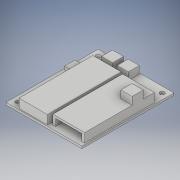
# Autodesk Inventor part: PCB
Saved by Autodesk Inventor 2017 (Build 210142000, 142)
## iProperties
Created: 2017-03-19
Part Number: PCB
Material: Generic
Document SubType Name: Modeling
Designer: Liam
Density: 1 g/cm^3
Appearance: Default
Author: Liam
Autodesk Inventor part; units mm, degrees
ref_plane "YZ Plane" through (0, 0, 0) normal (1, 0, 0) x (0, 1, 0)
ref_plane "XZ Plane" through (0, 0, 0) normal (0, 1, 0) x (-1, 0, 0)
ref_plane "XY Plane" through (0, 0, 0) normal (0, 0, 1) x (1, 0, 0)
sketch "Sketch1" plane through (0, 0, 0) normal (0, 1, 0) x (-1, 0, 0)
  line L0 (0, 0) -> (-54.5338, 0)
  line L1 (-54.5338, 0) -> (-54.5338, -66.1924)
  line L2 (-54.5338, -66.1924) -> (0, -66.1924)
  line L3 (0, -66.1924) -> (0, 0)
  dimension "d0" = 54.5338
  dimension "d1" = 66.1924
  constraints: 8 end point, 2 parallel, 1 horizontal, 1 perpendicular
  measures "d0" distance of L2.end L1.end
  measures "d1" distance of L1.end L0.end
extrude "Extrusion1" add sketch "Sketch1" along normal blind 1.5875
sketch "Sketch2" plane through (0, 1.5875, 0) normal (0, 1, 0) x (1, 0, 0)
  line L0 (0, 66.1924) -> (0, 0) projected
  line L1 (54.5338, 66.1924) -> (0, 66.1924) projected
  line L2 (54.5338, 0) -> (54.5338, 66.1924) projected
  line L3 (0, 0) -> (54.5338, 0) projected
  point P0 (4.3434, 61.7982)
  point P1 (50.419, 61.849)
  point P2 (4.0894, 4.4196)
  dimension "d4" = 4.3434
  dimension "d5" = 4.3942
  dimension "d6" = 4.1148
  dimension "d7" = 4.3434
  dimension "d8" = 4.0894
  dimension "d9" = 4.4196
  measures "d4" distance from line of L0 point (4.343, 61.798)
  measures "d5" distance from line of point (4.343, 61.798) L1
  measures "d6" distance from line of point (50.419, 61.849) L2
  measures "d7" distance from line of point (50.419, 61.849) L1
  measures "d8" distance from line of point (4.089, 4.42) L0
  measures "d9" distance from line of L3 point (4.089, 4.42)
hole "Hole1" at (4.3434, 1.5875, -61.7982) at (50.419, 1.5875, -61.849) at (4.0894, 1.5875, -4.4196) direction (0, -1, 0) diameter 3.175 end through all
sketch "Sketch3" plane through (0, 1.5875, 0) normal (0, 1, 0) x (1, 0, 0)
  line L0 (53.721, 52.8828) -> (53.721, 2.8448)
  line L1 (30.861, 2.8448) -> (30.861, 52.8828)
  line L2 (0, 0) -> (54.5338, 0) projected
  line L3 (54.5338, 0) -> (54.5338, 66.1924) projected
  line L4 (32.893, 52.8828) -> (32.893, 2.8448)
  line L5 (51.689, 52.8828) -> (51.689, 2.8448)
  line L6 (30.861, 52.8828) -> (32.893, 52.8828)
  line L7 (51.689, 52.8828) -> (53.721, 52.8828)
  line L8 (53.721, 2.8448) -> (51.689, 2.8448)
  line L9 (32.893, 2.8448) -> (30.861, 2.8448)
  dimension "d17" = 22.86
  dimension "d18" = 50.038
  dimension "d20" = 0.8128
  dimension "d21" = 2.032
  dimension "d22" = 2.032
  constraints: 16 end point, 6 perpendicular, 5 parallel, 2 horizontal
  measures "d17" distance of L0.end L1.start
  measures "d18" distance of L0.start L0.end
  measures "d20" distance between parallel lines of L3 L0
  measures "d21" distance between parallel lines of L4 L1
  measures "d22" distance between parallel lines of L5 L0
extrude "Extrusion2" add sketch "Sketch3" along normal blind 5
sketch "Sketch4" plane through (0, 6.5875, 0) normal (0, 1, 0) x (1, 0, 0)
  line L0 (30.861, 52.8828) -> (30.861, 2.8448) projected
  line L1 (30.861, 2.8448) -> (32.893, 2.8448) projected
  line L2 (32.893, 2.8448) -> (32.893, 52.8828) projected
  line L3 (32.893, 52.8828) -> (30.861, 52.8828) projected
  line L4 (53.721, 2.8448) -> (53.721, 52.8828) projected
  line L5 (51.689, 52.8828) -> (51.689, 2.8448) projected
  line L6 (51.689, 2.8448) -> (53.721, 2.8448) projected
  line L7 (53.721, 52.8828) -> (51.689, 52.8828) projected
  line L8 (30.861, 52.8828) -> (30.861, 2.8448) projected
  line L9 (30.861, 52.8828) -> (53.721, 52.8828)
  line L10 (53.721, 52.8828) -> (53.721, 2.8448)
  line L11 (53.721, 2.8448) -> (30.861, 2.8448)
  line L12 (30.861, 2.8448) -> (30.861, 52.8828)
  point P0 (0, 0)
  constraints: 8 end point, 2 parallel, 1 horizontal, 1 perpendicular
extrude "Extrusion3" add sketch "Sketch4" along normal blind 1.5875
sketch "Sketch5" plane through (0, 8.175, 0) normal (0, 1, 0) x (1, 0, 0)
  line L0 (45.721, 44.8828) -> (53.721, 44.8828)
  line L1 (53.721, 44.8828) -> (53.721, 36.8828)
  line L2 (53.721, 36.8828) -> (45.721, 36.8828)
  line L3 (45.721, 36.8828) -> (45.721, 44.8828)
  line L4 (53.721, 2.8448) -> (53.721, 52.8828) projected
  line L5 (53.721, 52.8828) -> (30.861, 52.8828) projected
  point P0 (0, 0)
  dimension "d27" = 8
  dimension "d28" = 8
  dimension "d29" = 8
  constraints: 8 end point, 2 collinear, 2 parallel, 1 horizontal, 1 perpendicular
  measures "d27" distance of L1.end L2.end
  measures "d28" distance of L0.end L1.end
  measures "d29" distance between parallel lines of L0 L5
extrude "Extrusion4" add sketch "Sketch5" along normal blind 5.5
sketch "Sketch7" plane through (0, 1.5875, 0) normal (0, 1, 0) x (1, 0, 0)
  line L0 (1.016, 48.7426) -> (6.096, 48.7426)
  line L1 (6.096, 48.7426) -> (6.096, 41.1226)
  line L2 (6.096, 41.1226) -> (1.016, 41.1226)
  line L3 (1.016, 41.1226) -> (1.016, 48.7426)
  line L4 (54.5338, 66.1924) -> (0, 66.1924) projected
  line L5 (0, 66.1924) -> (0, 0) projected
  dimension "d32" = 5.08
  dimension "d33" = 7.62
  dimension "d34" = 17.4498
  dimension "d35" = 1.016
  constraints: 8 end point, 2 parallel, 1 horizontal, 1 perpendicular
  measures "d32" distance of L1.end L2.end
  measures "d33" distance of L0.end L1.end
  measures "d34" distance between parallel lines of L0 L4
  measures "d35" distance between parallel lines of L5 L3
extrude "Extrusion5" add sketch "Sketch7" along normal blind 2.5
sketch "Sketch8" plane through (0, 1.5875, 0) normal (0, 1, 0) x (1, 0, 0)
  line L0 (11.2522, 65.3034) -> (19.2532, 65.3034)
  line L1 (19.2532, 65.3034) -> (19.2532, 57.3024)
  line L2 (19.2532, 57.3024) -> (11.2522, 57.3024)
  line L3 (11.2522, 57.3024) -> (11.2522, 65.3034)
  line L4 (0, 66.1924) -> (0, 0) projected
  line L5 (54.5338, 66.1924) -> (0, 66.1924) projected
  line L6 (22.5044, 65.3034) -> (30.5054, 65.3034)
  line L7 (30.5054, 65.3034) -> (30.5054, 57.3024)
  line L8 (30.5054, 57.3024) -> (22.5044, 57.3024)
  line L9 (22.5044, 57.3024) -> (22.5044, 65.3034)
  dimension "d38" = 8.001
  dimension "d39" = 8.001
  dimension "d40" = 11.2522
  dimension "d41" = 0.889
  dimension "d42" = 8.001
  dimension "d43" = 8.001
  dimension "d44" = 3.2512
  dimension "d45" = 0.889
  constraints: 16 end point, 4 parallel, 2 horizontal, 2 perpendicular
  measures "d38" distance of L1.end L2.end
  measures "d39" distance of L0.end L1.end
  measures "d40" distance between parallel lines of L3 L4
  measures "d41" distance between parallel lines of L0 L5
  measures "d42" distance of L7.end L8.end
  measures "d43" distance of L6.end L7.end
  measures "d44" distance between parallel lines of L9 L1
  measures "d45" distance between parallel lines of L6 L5
extrude "Extrusion6" add sketch "Sketch8" along normal blind 5.5
sketch "Sketch9" plane through (0, 1.5875, 0) normal (0, 1, 0) x (1, 0, 0)
  line L0 (8.6868, 53.7464) -> (29.0322, 53.7464)
  line L1 (29.0322, 53.7464) -> (29.0322, 0.6858)
  line L2 (29.0322, 0.6858) -> (8.6868, 0.6858)
  line L3 (8.6868, 0.6858) -> (8.6868, 53.7464)
  line L4 (54.5338, 66.1924) -> (0, 66.1924) projected
  line L5 (30.861, 52.8828) -> (30.861, 2.8448) projected
  line L6 (0, 66.1924) -> (0, 0) projected
  line L7 (0, 0) -> (54.5338, 0) projected
  dimension "d48" = 12.446
  dimension "d49" = 1.8288
  dimension "d50" = 8.6868
  dimension "d51" = 0.6858
  constraints: 8 end point, 2 parallel, 1 horizontal, 1 perpendicular
  measures "d48" distance between parallel lines of L0 L4
  measures "d49" distance between parallel lines of L5 L1
  measures "d50" distance between parallel lines of L6 L3
  measures "d51" distance between parallel lines of L7 L2
extrude "Extrusion7" add sketch "Sketch9" along normal up to surface (6.5875 mm away)
sketch "Sketch10" plane through (0, 0, 0) normal (0, -1, 0) x (1, 0, 0)
  line L0 (42.7736, -21.8694) -> (24.1808, -21.8694)
  line L1 (24.1808, -21.8694) -> (24.1808, -12.2936)
  line L2 (24.1808, -12.2936) -> (42.7736, -12.2936)
  line L3 (42.7736, -12.2936) -> (42.7736, -21.8694)
  line L4 (54.5338, -66.1924) -> (0, -66.1924) projected
  line L5 (54.5338, 0) -> (54.5338, -66.1924) projected
  line L6 (0, -66.1924) -> (0, 0) projected
  line L7 (0, 0) -> (54.5338, 0) projected
  dimension "d54" = 44.323
  dimension "d55" = 11.7602
  dimension "d56" = 24.1808
  dimension "d57" = 12.2936
  constraints: 8 end point, 2 parallel, 1 horizontal, 1 perpendicular
  measures "d54" distance between parallel lines of L4 L0
  measures "d55" distance between parallel lines of L5 L3
  measures "d56" distance between parallel lines of L6 L1
  measures "d57" distance between parallel lines of L2 L7
extrude "Extrusion8" add sketch "Sketch10" along normal blind 1.016 contours L0 L1 L2 L3
body "Solid1"
